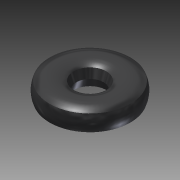
# Autodesk Inventor part: tire
Saved by Autodesk Inventor 2013 (Build 170138000, 138)
## iProperties
Created: 2013-07-22
Part Number: tire
Material: Generic
Document SubType Name: Modeling
Designer: dkboone
Density: 1 g/cm^3
Author: dkboone
Autodesk Inventor part; units mm, degrees
ref_plane "YZ Plane" through (0, 0, 0) normal (1, 0, 0) x (0, 1, 0)
ref_plane "XZ Plane" through (0, 0, 0) normal (0, 1, 0) x (-1, 0, 0)
ref_plane "XY Plane" through (0, 0, 0) normal (0, 0, 1) x (1, 0, 0)
sketch "Sketch1" plane through (0, 0, 0) normal (1, 0, 0) x (0, 1, 0)
  line L0 (0, 0) -> (0, 24.6063) construction
  arc A0 (-4.7625, 23.622) -> (-4.7625, 9.525) centre (5.802, 16.5735) ccw
  line L1 (-4.7625, 9.525) -> (0, 7.9375)
  line L2 (-9.6572, 0) -> (9.6572, 0) projected
  arc A1 (0, 24.6063) -> (-4.7625, 23.622) centre (0, 12.5919) ccw
  arc A2 (4.7625, 9.525) -> (4.7625, 23.622) centre (-5.802, 16.5735) ccw
  line L3 (4.7625, 9.525) -> (0, 7.9375)
  arc A3 (4.7625, 23.622) -> (0, 24.6063) centre (0, 12.5919) ccw
  dimension "d1" = 9.525
  dimension "d2" = 7.9375
  dimension "d4" = 4.7625
  dimension "d5" = 12.7
  dimension "d7" = 24.6062
  dimension "d8" = 4.7625
  dimension "d9" = 23.622
  constraints: 8 point on circle, 6 end point, 4 centre point, 3 symmetric about line, 2 point on line, 1 vertical, 2 other
  measures "d1" vertical distance of L1.start L0.start
  measures "d2" distance of L1.end L0.start
  measures "d4" horizontal distance of L0.start L1.start
  measures "d5" radius of A0
  measures "d7" distance of L0.start L0.end
  measures "d8" horizontal distance of A0.start L0.end
  measures "d9" vertical distance of L0.start A0.start
revolve "Revolution1" add sketch "Sketch1" angle 360 about axis through (0, -10, 0) along (0, 1, 0)
body "Solid1"
